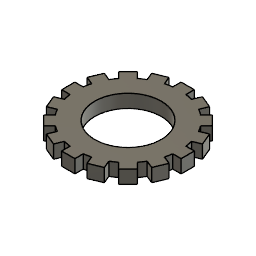
29aug2 (Autodesk Fusion 360 design; units mm, degrees)
part number: 2026-08-29-10-35-58-501
Autodesk Fusion 360 part; units mm, degrees
sketch "Sketch1" plane through (0, 0, 0) normal (0, 1, 0) x (1, 0, 0)
  circle A0 centre (0, 0) radius 25
  circle A1 centre (0, 0) radius 39
  line L0 (5, 45) -> (-5, 45)
  line L1 (-5, -45) -> (5, -45)
  line L2 (-5, 45) -> (-5, 38.6782)
  line L3 (-5, -38.6782) -> (-5, -45)
  line L4 (-5, 45) -> (-4.9694, 44.7248) construction
  line L5 (4.9694, -44.7248) -> (5, -45) construction
  line L6 (5, 45) -> (4.9694, 44.7248) construction
  line L7 (-4.9694, -44.7248) -> (-5, -45) construction
  line L8 (5, -45) -> (5, -38.6782)
  line L9 (5, 38.6782) -> (5, 45)
  line L10 (-10.1821, 37.6474) -> (-12.6014, 43.488)
  line L11 (-12.6014, 43.488) -> (-21.8402, 39.6612)
  line L12 (-21.8402, 39.6612) -> (-19.4209, 33.8205)
  line L13 (21.8402, -39.6612) -> (19.4209, -33.8205)
  line L14 (12.6014, -43.488) -> (21.8402, -39.6612)
  line L15 (10.1821, -37.6474) -> (12.6014, -43.488)
  line L16 (-23.8141, 30.8851) -> (-28.2843, 35.3553)
  line L17 (-28.2843, 35.3553) -> (-35.3553, 28.2843)
  line L18 (-35.3553, 28.2843) -> (-30.8851, 23.8141)
  line L19 (35.3553, -28.2843) -> (30.8851, -23.8141)
  line L20 (28.2843, -35.3553) -> (35.3553, -28.2843)
  line L21 (23.8141, -30.8851) -> (28.2843, -35.3553)
  line L22 (-33.8205, 19.4209) -> (-39.6612, 21.8402)
  line L23 (-39.6612, 21.8402) -> (-43.488, 12.6014)
  line L24 (-43.488, 12.6014) -> (-37.6474, 10.1821)
  line L25 (43.488, -12.6014) -> (37.6474, -10.1821)
  line L26 (39.6612, -21.8402) -> (43.488, -12.6014)
  line L27 (33.8205, -19.4209) -> (39.6612, -21.8402)
  line L28 (-38.6782, 5) -> (-45, 5)
  line L29 (-45, 5) -> (-45, -5)
  line L30 (-45, -5) -> (-38.6782, -5)
  line L31 (45, 5) -> (38.6782, 5)
  line L32 (45, -5) -> (45, 5)
  line L33 (38.6782, -5) -> (45, -5)
  line L34 (-37.6474, -10.1821) -> (-43.488, -12.6014)
  line L35 (-43.488, -12.6014) -> (-39.6612, -21.8402)
  line L36 (-39.6612, -21.8402) -> (-33.8205, -19.4209)
  line L37 (39.6612, 21.8402) -> (33.8205, 19.4209)
  line L38 (43.488, 12.6014) -> (39.6612, 21.8402)
  line L39 (37.6474, 10.1821) -> (43.488, 12.6014)
  line L40 (-30.8851, -23.8141) -> (-35.3553, -28.2843)
  line L41 (-35.3553, -28.2843) -> (-28.2843, -35.3553)
  line L42 (-28.2843, -35.3553) -> (-23.8141, -30.8851)
  line L43 (28.2843, 35.3553) -> (23.8141, 30.8851)
  line L44 (35.3553, 28.2843) -> (28.2843, 35.3553)
  line L45 (30.8851, 23.8141) -> (35.3553, 28.2843)
  line L46 (-19.4209, -33.8205) -> (-21.8402, -39.6612)
  line L47 (-21.8402, -39.6612) -> (-12.6014, -43.488)
  line L48 (-12.6014, -43.488) -> (-10.1821, -37.6474)
  line L49 (12.6014, 43.488) -> (10.1821, 37.6474)
  line L50 (21.8402, 39.6612) -> (12.6014, 43.488)
  line L51 (19.4209, 33.8205) -> (21.8402, 39.6612)
  line L52 (-5, -38.6782) -> (-5, -45)
  line L53 (-5, -45) -> (5, -45)
  line L54 (5, -45) -> (5, -38.6782)
  line L55 (-5, 45) -> (-5, 38.6782)
  line L56 (5, 45) -> (-5, 45)
  line L57 (5, 38.6782) -> (5, 45)
  line L58 (10.1821, -37.6474) -> (12.6014, -43.488)
  line L59 (12.6014, -43.488) -> (21.8402, -39.6612)
  line L60 (21.8402, -39.6612) -> (19.4209, -33.8205)
  line L61 (-21.8402, 39.6612) -> (-19.4209, 33.8205)
  line L62 (-12.6014, 43.488) -> (-21.8402, 39.6612)
  line L63 (-10.1821, 37.6474) -> (-12.6014, 43.488)
  line L64 (23.8141, -30.8851) -> (28.2843, -35.3553)
  line L65 (28.2843, -35.3553) -> (35.3553, -28.2843)
  line L66 (35.3553, -28.2843) -> (30.8851, -23.8141)
  line L67 (-35.3553, 28.2843) -> (-30.8851, 23.8141)
  line L68 (-28.2843, 35.3553) -> (-35.3553, 28.2843)
  line L69 (-23.8141, 30.8851) -> (-28.2843, 35.3553)
  line L70 (33.8205, -19.4209) -> (39.6612, -21.8402)
  line L71 (39.6612, -21.8402) -> (43.488, -12.6014)
  line L72 (43.488, -12.6014) -> (37.6474, -10.1821)
  line L73 (-43.488, 12.6014) -> (-37.6474, 10.1821)
  line L74 (-39.6612, 21.8402) -> (-43.488, 12.6014)
  line L75 (-33.8205, 19.4209) -> (-39.6612, 21.8402)
  line L76 (38.6782, -5) -> (45, -5)
  line L77 (45, -5) -> (45, 5)
  line L78 (45, 5) -> (38.6782, 5)
  line L79 (-45, -5) -> (-38.6782, -5)
  line L80 (-45, 5) -> (-45, -5)
  line L81 (-38.6782, 5) -> (-45, 5)
  line L82 (37.6474, 10.1821) -> (43.488, 12.6014)
  line L83 (43.488, 12.6014) -> (39.6612, 21.8402)
  line L84 (39.6612, 21.8402) -> (33.8205, 19.4209)
  line L85 (-39.6612, -21.8402) -> (-33.8205, -19.4209)
  line L86 (-43.488, -12.6014) -> (-39.6612, -21.8402)
  line L87 (-37.6474, -10.1821) -> (-43.488, -12.6014)
  line L88 (30.8851, 23.8141) -> (35.3553, 28.2843)
  line L89 (35.3553, 28.2843) -> (28.2843, 35.3553)
  line L90 (28.2843, 35.3553) -> (23.8141, 30.8851)
  line L91 (-28.2843, -35.3553) -> (-23.8141, -30.8851)
  line L92 (-35.3553, -28.2843) -> (-28.2843, -35.3553)
  line L93 (-30.8851, -23.8141) -> (-35.3553, -28.2843)
  line L94 (19.4209, 33.8205) -> (21.8402, 39.6612)
  line L95 (21.8402, 39.6612) -> (12.6014, 43.488)
  line L96 (12.6014, 43.488) -> (10.1821, 37.6474)
  line L97 (-12.6014, -43.488) -> (-10.1821, -37.6474)
  line L98 (-21.8402, -39.6612) -> (-12.6014, -43.488)
  line L99 (-19.4209, -33.8205) -> (-21.8402, -39.6612)
  dimension "d1" = 50
  dimension "d3" = 78
  dimension "d4" = 10
  dimension "d5" = 90
  dimension "d7" = 360
  constraint coincident A0.centre A1.centre
  constraint concentric A0 A1
  constraint horizontal L0
  constraint perpendicular L0 L2
  constraint parallel L0 L1
  constraint parallel L2 L9
  constraint coincident A0.centre L7
  constraint coincident A0.centre L5
  constraint coincident A1 L2.end
  constraint collinear L2 L3
  constraint collinear L4 L5
  constraint collinear L6 L7
  constraint coincident A1 L9.start
  constraint collinear L8 L9
  constraint coincident A1 L8.end
  constraint coincident A1 L3.start
  measures "d1" diameter of A0
  measures "d3" diameter of A1
  measures "d4" distance of L1.start L1.end
  measures "d5" distance of L0.end L1.start
extrude "Extrude1" add sketch "Sketch1" along normal blind 10
